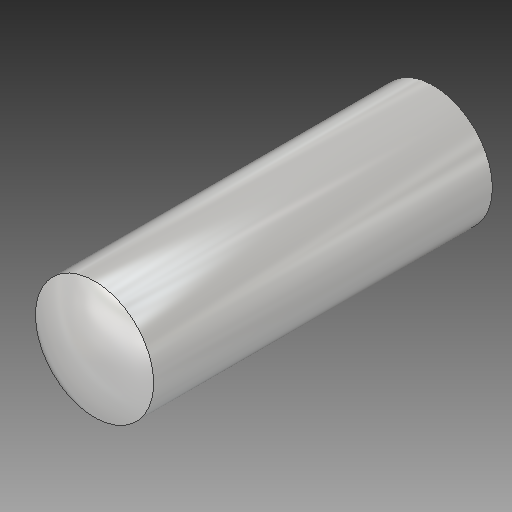
# Autodesk Inventor part: idler bearing pin
Saved by Autodesk Inventor 2018 (Build 220112000, 112)
## iProperties
Created: 2016-06-27
Part Number: idler bearing pin
Material: Generic
Document SubType Name: Modeling
Designer: Ben
Density: 1 g/cm^3
Appearance: Default
Author: Ben
Autodesk Inventor part; units mm, degrees
ref_plane "YZ Plane" through (0, 0, 0) normal (1, 0, 0) x (0, 1, 0)
ref_plane "XZ Plane" through (0, 0, 0) normal (0, 1, 0) x (-1, 0, 0)
ref_plane "XY Plane" through (0, 0, 0) normal (0, 0, 1) x (1, 0, 0)
sketch "Sketch1" plane through (0, 0, 0) normal (0, 0, 1) x (1, 0, 0)
  circle A0 centre (0, 0) radius 1.5
  dimension "d0" = 3
  constraints: 1 centre point, 1 coincident
  measures "d0" diameter of A0
extrude "Extrusion1" add sketch "Sketch1" along normal blind 9
sketch "Sketch2" plane through (0, 0, 0) normal (0, 1, 0) x (-1, 0, 0)
  line L0 (1.5, 9) -> (-1.5, 9) projected
  line L1 (0, 0) -> (0, 10.4937) construction
  line L2 (1.5, 0) -> (1.5, 9) projected
  line L3 (-1.5, 0) -> (-1.5, 9) projected
  arc A0 (1.5, 8.5981) -> (0, 9) centre (0, 6) ccw
  arc A1 (-1.5, 3.4019) -> (1.5, 3.4019) centre (0, 6) ccw
  line L4 (0, 9) -> (1.5, 9)
  line L5 (1.5, 9) -> (1.5, 8.5981)
  dimension "d4" = 3
  constraints: 6 end point, 5 point on line, 4 point on circle, 2 centre point, 2 tangent, 2 vertical, 1 collinear
  measures "d4" radius of A0
revolve "Revolution1" cut sketch "Sketch2" angle 360 about axis through (0, 0, 0) along (0, 0, 1) contours L2 A0 L0
body "Solid1"
